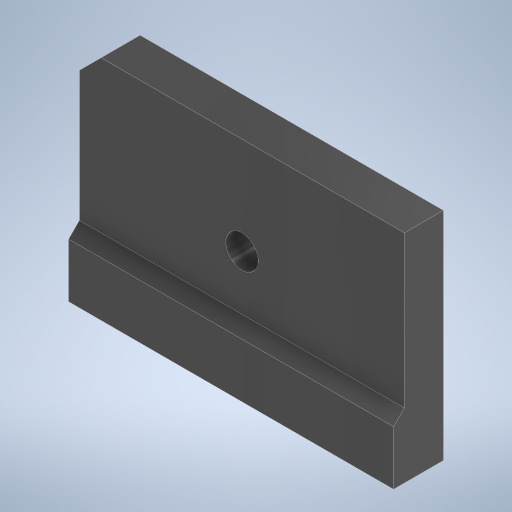
# Autodesk Inventor part: BrueckenGR_LVE2560E
Saved by Autodesk Inventor 2023.1 (Build 271208000, 208)
## iProperties
Created: 2023-11-19
Part Number: BrueckenGR_LVE2560E
Material: Generic
Document SubType Name: Modeling
Designer: JansenL
Density: 1 g/cm^3
Appearance: Dark Gray
Author: JansenL
Autodesk Inventor part; units mm, degrees
ref_plane "YZ Plane" through (0, 0, 0) normal (1, 0, 0) x (0, 1, 0)
ref_plane "XZ Plane" through (0, 0, 0) normal (0, 1, 0) x (-1, 0, 0)
ref_plane "XY Plane" through (0, 0, 0) normal (0, 0, 1) x (1, 0, 0)
sketch "Sketch1" plane through (0, 0, 0) normal (1, 0, 0) x (0, 1, 0)
  line L0 (0, 0) -> (0, -4.6)
  line L1 (0, -4.6) -> (20, -4.6)
  line L2 (20, -4.6) -> (20, -1)
  line L3 (20, -1) -> (6, -1)
  line L4 (6, -1) -> (5, 0)
  line L5 (5, 0) -> (0, 0)
  dimension "d1" = 20
  dimension "d2" = 5
  dimension "d3" = 3.6
  dimension "d4" = 4.6
  dimension "d5" = 1
  constraints: 12 end point, 3 perpendicular, 1 coincident, 1 parallel, 1 vertical
  measures "d1" distance of L0.end L1.end
  measures "d2" distance of L4.end L0.start
  measures "d3" distance between parallel lines of L1 L3
  measures "d4" distance between parallel lines of L1 L5
  measures "d5" horizontal distance of L3.end L4.end
extrude "Extrusion1" add sketch "Sketch1" along normal blind 30
chamfer "Chamfer1" distance 2 angle 45 1 edges at (0, 20, -2.8)
sketch "Sketch2" plane through (0, 6, -1) normal (0, 0, 1) x (1, 0, 0)
  circle A0 centre (15, 5) radius 1.6
  line L0 (0, -6) -> (30, -6) projected
  line L1 (30, 14) -> (30, 0) projected
  dimension "d11" = 11
  dimension "d12" = 3.2
  dimension "d13" = 15
  constraints: 1 centre point
  measures "d11" distance from line of L0 A0.centre
  measures "d12" diameter of A0
  measures "d13" distance from line of L1 A0.centre
hole "Hole1" at (15, 11, -1) direction (0, 0, -1) diameter 3 depth 10 tip angle 118
body "Solid1"
